Autodesk Inventor part; units mm, degrees
(part 2 of 3)
  line L936 (44.1495, 7.0872) -> (44.0754, 6.988)
  line L937 (44.0754, 6.988) -> (43.9994, 6.8902)
  line L938 (43.9994, 6.8902) -> (43.7335, 6.2149)
  line L939 (43.7335, 6.2149) -> (43.6108, 5.2944)
  line L940 (43.6108, 5.2944) -> (43.608, 5.0726)
  line L941 (43.608, 5.0726) -> (42.6667, 5.0726)
  line L942 (42.6667, 5.0726) -> (42.6667, 8.4846)
  line L943 (42.6667, 8.4846) -> (50.4254, 8.4846)
  line L944 (50.4254, 8.4846) -> (50.4254, 5.0726)
  line L945 (50.4254, 5.0726) -> (49.484, 5.0726)
  line L946 (49.484, 5.0726) -> (49.4812, 5.2903)
  line L947 (49.4812, 5.2903) -> (49.3613, 6.2039)
  line L948 (49.3613, 6.2039) -> (49.0967, 6.8806)
  line L949 (49.0967, 6.8806) -> (49.0223, 6.9798)
  line L950 (49.0223, 6.9798) -> (48.9466, 7.0804)
  line L951 (48.9466, 7.0804) -> (48.4381, 7.429)
  line L952 (48.4381, 7.429) -> (47.8013, 7.5792)
  line L953 (47.8013, 7.5792) -> (47.5889, 7.5792)
  line L954 (47.5889, 7.5792) -> (47.4088, 7.5792)
  line L955 (47.4088, 7.5792) -> (47.4088, 1.943)
  line L956 (47.4088, 1.943) -> (47.4088, 1.7859)
  line L957 (47.4088, 1.7859) -> (47.5204, 1.3353)
  line L958 (47.5204, 1.3353) -> (47.544, 1.3133)
  line L959 (47.544, 1.3133) -> (47.5658, 1.2912)
  line L960 (47.5658, 1.2912) -> (48.0631, 1.181)
  line L961 (48.0631, 1.181) -> (48.23, 1.181)
  line L962 (48.23, 1.181) -> (48.9313, 1.181)
  line L963 (48.9313, 1.181) -> (48.9313, 0.2453)
  line L964 (48.9313, 0.2453) -> (44.1536, 0.2453)
  line L965 (44.1536, 0.2453) -> (44.1536, 1.181)
  line L966 (44.1536, 1.181) -> (44.8663, 1.181)
  line L967 (44.8663, 1.181) -> (45.0357, 1.181)
  line L968 (45.0357, 1.181) -> (45.5221, 1.2898)
  line L969 (45.5221, 1.2898) -> (45.5442, 1.3105)
  line L970 (45.5442, 1.3105) -> (45.5661, 1.3326)
  line L971 (45.5661, 1.3326) -> (45.6766, 1.7915)
  line L972 (45.6766, 1.7915) -> (45.6766, 1.943)
  line L973 (45.6766, 1.943) -> (45.6766, 7.5792)
  line L974 (52.4548, 0.2453) -> (52.4548, 1.181)
  line L975 (52.4548, 1.181) -> (52.9361, 1.181)
  line L976 (52.9361, 1.181) -> (53.104, 1.181)
  line L977 (53.104, 1.181) -> (53.5904, 1.2898)
  line L978 (53.5904, 1.2898) -> (53.6128, 1.3105)
  line L979 (53.6128, 1.3105) -> (53.6346, 1.3326)
  line L980 (53.6346, 1.3326) -> (53.7449, 1.7915)
  line L981 (53.7449, 1.7915) -> (53.7449, 1.943)
  line L982 (53.7449, 1.943) -> (53.7449, 6.7937)
  line L983 (53.7449, 6.7937) -> (53.7449, 6.9522)
  line L984 (53.7449, 6.9522) -> (53.6346, 7.4056)
  line L985 (53.6346, 7.4056) -> (53.6128, 7.4262)
  line L986 (53.6128, 7.4262) -> (53.5904, 7.4483)
  line L987 (53.5904, 7.4483) -> (53.0987, 7.5544)
  line L988 (53.0987, 7.5544) -> (52.9361, 7.5544)
  line L989 (52.9361, 7.5544) -> (52.4548, 7.5544)
  line L990 (52.4548, 7.5544) -> (52.4548, 8.4846)
  line L991 (52.4548, 8.4846) -> (60.5618, 8.4846)
  line L992 (60.5618, 8.4846) -> (60.5618, 5.2047)
  line L993 (60.5618, 5.2047) -> (59.6263, 5.2047)
  line L994 (59.6263, 5.2047) -> (59.6192, 5.4403)
  line L995 (59.6192, 5.4403) -> (59.494, 6.3788)
  line L996 (59.494, 6.3788) -> (59.2375, 7.0058)
  line L997 (59.2375, 7.0058) -> (59.1674, 7.0843)
  line L998 (59.1674, 7.0843) -> (59.0973, 7.1629)
  line L999 (59.0973, 7.1629) -> (58.5278, 7.4371)
  line L1000 (58.5278, 7.4371) -> (57.7231, 7.5543)
  line L1001 (57.7231, 7.5543) -> (57.4557, 7.5543)
  line L1002 (57.4557, 7.5543) -> (55.477, 7.5543)
  line L1003 (55.477, 7.5543) -> (55.477, 5.0242)
  line L1004 (55.477, 5.0242) -> (55.9454, 5.0242)
  line L1005 (55.9454, 5.0242) -> (56.1054, 5.0242)
  line L1006 (56.1054, 5.0242) -> (56.5847, 5.0917)
  line L1007 (56.5847, 5.0917) -> (56.9184, 5.2474)
  line L1008 (56.9184, 5.2474) -> (56.9583, 5.2915)
  line L1009 (56.9583, 5.2915) -> (56.9982, 5.337)
  line L1010 (56.9982, 5.337) -> (57.1526, 5.7311)
  line L1011 (57.1526, 5.7311) -> (57.2476, 6.3581)
  line L1012 (57.2476, 6.3581) -> (57.2588, 6.518)
  line L1013 (57.2588, 6.518) -> (58.193, 6.5235)
  line L1014 (58.193, 6.5235) -> (58.193, 2.3921)
  line L1015 (58.193, 2.3921) -> (57.2588, 2.399)
  line L1016 (57.2588, 2.399) -> (57.2489, 2.5768)
  line L1017 (57.2489, 2.5768) -> (57.1569, 3.2727)
  line L1018 (57.1569, 3.2727) -> (57.0038, 3.7178)
  line L1019 (57.0038, 3.7178) -> (56.9639, 3.7688)
  line L1020 (56.9639, 3.7688) -> (56.9238, 3.8211)
  line L1021 (56.9238, 3.8211) -> (56.5918, 4.0003)
  line L1022 (56.5918, 4.0003) -> (56.1148, 4.0775)
  line L1023 (56.1148, 4.0775) -> (55.9563, 4.0775)
  line L1024 (55.9563, 4.0775) -> (55.477, 4.0775)
  line L1025 (55.477, 4.0775) -> (55.477, 1.1808)
  line L1026 (55.477, 1.1808) -> (57.6362, 1.1808)
  line L1027 (57.6362, 1.1808) -> (57.8636, 1.1808)
  line L1028 (57.8636, 1.1808) -> (58.5458, 1.3062)
  line L1029 (58.5458, 1.3062) -> (59.0487, 1.5998)
  line L1030 (59.0487, 1.5998) -> (59.1163, 1.6825)
  line L1031 (59.1163, 1.6825) -> (59.1826, 1.7665)
  line L1032 (59.1826, 1.7665) -> (59.4442, 2.4459)
  line L1033 (59.4442, 2.4459) -> (59.6083, 3.4767)
  line L1034 (59.6083, 3.4767) -> (59.6263, 3.7357)
  line L1035 (59.6263, 3.7357) -> (60.562, 3.7357)
  line L1036 (60.562, 3.7357) -> (60.562, 0.2453)
  line L1037 (60.562, 0.2453) -> (52.4548, 0.2453)
  line L1038 (69.1459, 3.4353) -> (70.2, 3.4353)
  line L1039 (70.2, 3.4353) -> (70.1798, 3.1625)
  line L1040 (70.1798, 3.1625) -> (69.8872, 1.9801)
  line L1041 (69.8872, 1.9801) -> (69.3375, 1.0459)
  line L1042 (69.3375, 1.0459) -> (69.1899, 0.8957)
  line L1043 (69.1899, 0.8957) -> (69.041, 0.7469)
  line L1044 (69.041, 0.7469) -> (68.1426, 0.2246)
  line L1045 (68.1426, 0.2246) -> (67.1215, 0)
  line L1046 (67.1215, 0) -> (66.7827, 0)
  line L1047 (66.7827, 0) -> (66.3735, 0)
  line L1048 (66.3735, 0) -> (65.2668, 0.2356)
  line L1049 (65.2668, 0.2356) -> (65.1454, 0.2825)
  line L1050 (65.1454, 0.2825) -> (65.0225, 0.3294)
  line L1051 (65.0225, 0.3294) -> (63.9338, 1.0487)
  line L1052 (63.9338, 1.0487) -> (63.8391, 1.1451)
  line L1053 (63.8391, 1.1451) -> (63.7329, 1.2513)
  line L1054 (63.7329, 1.2513) -> (62.931, 2.4626)
  line L1055 (62.931, 2.4626) -> (62.8769, 2.599)
  line L1056 (62.8769, 2.599) -> (62.8221, 2.7368)
  line L1057 (62.8221, 2.7368) -> (62.5508, 3.9632)
  line L1058 (62.5508, 3.9632) -> (62.5508, 4.3711)
  line L1059 (62.5508, 4.3711) -> (62.5508, 4.808)
  line L1060 (62.5508, 4.808) -> (62.8139, 5.9862)
  line L1061 (62.8139, 5.9862) -> (62.8675, 6.1185)
  line L1062 (62.8675, 6.1185) -> (62.9196, 6.2522)
  line L1063 (62.9196, 6.2522) -> (63.7192, 7.4483)
  line L1064 (63.7192, 7.4483) -> (63.8266, 7.5544)
  line L1065 (63.8266, 7.5544) -> (63.9229, 7.6522)
  line L1066 (63.9229, 7.6522) -> (65.0075, 8.384)
  line L1067 (65.0075, 8.384) -> (65.1274, 8.4336)
  line L1068 (65.1274, 8.4336) -> (65.2473, 8.4832)
  line L1069 (65.2473, 8.4832) -> (66.3179, 8.7299)
  line L1070 (66.3179, 8.7299) -> (66.675, 8.7299)
  line L1071 (66.675, 8.7299) -> (66.9851, 8.7299)
  line L1072 (66.9851, 8.7299) -> (67.8216, 8.5576)
  line L1073 (67.8216, 8.5576) -> (67.9193, 8.5232)
  line L1074 (67.9193, 8.5232) -> (68.0159, 8.4887)
  line L1075 (68.0159, 8.4887) -> (68.9737, 7.9568)
  line L1076 (68.9737, 7.9568) -> (69.0672, 7.8852)
  line L1077 (69.0672, 7.8852) -> (69.3128, 8.6224)
  line L1078 (69.3128, 8.6224) -> (70.2, 8.6224)
  line L1079 (70.2, 8.6224) -> (70.2, 5.2461)
  line L1080 (70.2, 5.2461) -> (69.2533, 5.2461)
  line L1081 (69.2533, 5.2461) -> (69.2284, 5.4431)
  line L1082 (69.2284, 5.4431) -> (68.9912, 6.2948)
  line L1083 (68.9912, 6.2948) -> (68.5959, 6.9672)
  line L1084 (68.5959, 6.9672) -> (68.4938, 7.0747)
  line L1085 (68.4938, 7.0747) -> (68.3905, 7.1836)
  line L1086 (68.3905, 7.1836) -> (67.7897, 7.5612)
  line L1087 (67.7897, 7.5612) -> (67.1283, 7.7224)
  line L1088 (67.1283, 7.7224) -> (66.9091, 7.7224)
  line L1089 (66.9091, 7.7224) -> (66.6556, 7.7224)
  line L1090 (66.6556, 7.7224) -> (65.8977, 7.4964)
  line L1091 (65.8977, 7.4964) -> (65.2378, 6.9686)
  line L1092 (65.2378, 6.9686) -> (65.1316, 6.817)
  line L1093 (65.1316, 6.817) -> (65.0239, 6.6668)
  line L1094 (65.0239, 6.6668) -> (64.6478, 5.738)
  line L1095 (64.6478, 5.738) -> (64.4867, 4.6673)
  line L1096 (64.4867, 4.6673) -> (64.4867, 4.3104)
  line L1097 (64.4867, 4.3104) -> (64.4867, 3.9741)
  line L1098 (64.4867, 3.9741) -> (64.6465, 2.9613)
  line L1099 (64.6465, 2.9613) -> (65.0202, 2.0972)
  line L1100 (65.0202, 2.0972) -> (65.1273, 1.9581)
  line L1101 (65.1273, 1.9581) -> (65.2335, 1.8203)
  line L1102 (65.2335, 1.8203) -> (65.8992, 1.3352)
  line L1103 (65.8992, 1.3352) -> (66.6734, 1.1271)
  line L1104 (66.6734, 1.1271) -> (66.9325, 1.1271)
  line L1105 (66.9325, 1.1271) -> (67.1367, 1.1271)
  line L1106 (67.1367, 1.1271) -> (67.7512, 1.2759)
  line L1107 (67.7512, 1.2759) -> (68.3067, 1.6204)
  line L1108 (68.3067, 1.6204) -> (68.4019, 1.7183)
  line L1109 (68.4019, 1.7183) -> (68.4954, 1.8175)
  line L1110 (68.4954, 1.8175) -> (68.8688, 2.4431)
  line L1111 (68.8688, 2.4431) -> (69.1154, 3.2479)
  line L1112 (69.1154, 3.2479) -> (69.1459, 3.4353)
  line L1113 (71.6716, 0.2452) -> (71.6716, 1.1809)
  line L1114 (71.6716, 1.1809) -> (72.1512, 1.1809)
  line L1115 (72.1512, 1.1809) -> (72.3193, 1.1809)
  line L1116 (72.3193, 1.1809) -> (72.8057, 1.2897)
  line L1117 (72.8057, 1.2897) -> (72.8278, 1.3104)
  line L1118 (72.8278, 1.3104) -> (72.8499, 1.3325)
  line L1119 (72.8499, 1.3325) -> (72.9599, 1.7914)
  line L1120 (72.9599, 1.7914) -> (72.9599, 1.9429)
  line L1121 (72.9599, 1.9429) -> (72.9599, 6.7936)
  line L1122 (72.9599, 6.7936) -> (72.9599, 6.9521)
  line L1123 (72.9599, 6.9521) -> (72.8499, 7.4055)
  line L1124 (72.8499, 7.4055) -> (72.8278, 7.4262)
  line L1125 (72.8278, 7.4262) -> (72.8058, 7.4482)
  line L1126 (72.8058, 7.4482) -> (72.3138, 7.5543)
  line L1127 (72.3138, 7.5543) -> (72.1512, 7.5543)
  line L1128 (72.1512, 7.5543) -> (71.6716, 7.5543)
  line L1129 (71.6716, 7.5543) -> (71.6716, 8.4845)
  line L1130 (71.6716, 8.4845) -> (76.09, 8.4845)
  line L1131 (76.09, 8.4845) -> (76.09, 7.5543)
  line L1132 (76.09, 7.5543) -> (75.5152, 7.5543)
  line L1133 (75.5152, 7.5543) -> (75.3427, 7.5543)
  line L1134 (75.3427, 7.5543) -> (74.8494, 7.4441)
  line L1135 (74.8494, 7.4441) -> (74.8273, 7.4221)
  line L1136 (74.8273, 7.4221) -> (74.804, 7.4014)
  line L1137 (74.804, 7.4014) -> (74.6935, 6.9466)
  line L1138 (74.6935, 6.9466) -> (74.6935, 6.7936)
  line L1139 (74.6935, 6.7936) -> (74.6935, 4.9705)
  line L1140 (74.6935, 4.9705) -> (78.2546, 4.9705)
  line L1141 (78.2546, 4.9705) -> (78.2546, 6.7936)
  line L1142 (78.2546, 6.7936) -> (78.2546, 6.9521)
  line L1143 (78.2546, 6.9521) -> (78.1446, 7.4055)
  line L1144 (78.1446, 7.4055) -> (78.1223, 7.4262)
  line L1145 (78.1223, 7.4262) -> (78.1005, 7.4482)
  line L1146 (78.1005, 7.4482) -> (77.6082, 7.5543)
  line L1147 (77.6082, 7.5543) -> (77.4456, 7.5543)
  line L1148 (77.4456, 7.5543) -> (76.8642, 7.5543)
  line L1149 (76.8642, 7.5543) -> (76.8642, 8.4845)
  line L1150 (76.8642, 8.4845) -> (81.2889, 8.4845)
  line L1151 (81.2889, 8.4845) -> (81.2889, 7.5545)
  line L1152 (81.2889, 7.5545) -> (80.8081, 7.5545)
  line L1153 (80.8081, 7.5545) -> (80.6357, 7.5545)
  line L1154 (80.6357, 7.5545) -> (80.1439, 7.4443)
  line L1155 (80.1439, 7.4443) -> (80.1216, 7.4222)
  line L1156 (80.1216, 7.4222) -> (80.0984, 7.4016)
  line L1157 (80.0984, 7.4016) -> (79.9864, 6.9468)
  line L1158 (79.9864, 6.9468) -> (79.9864, 6.7938)
  line L1159 (79.9864, 6.7938) -> (79.9864, 1.9431)
  line L1160 (79.9864, 1.9431) -> (79.9864, 1.786)
  line L1161 (79.9864, 1.786) -> (80.0984, 1.3354)
  line L1162 (80.0984, 1.3354) -> (80.1215, 1.3134)
  line L1163 (80.1215, 1.3134) -> (80.1439, 1.2913)
  line L1164 (80.1439, 1.2913) -> (80.6412, 1.1811)
  line L1165 (80.6412, 1.1811) -> (80.8081, 1.1811)
  line L1166 (80.8081, 1.1811) -> (81.2885, 1.1811)
  line L1167 (81.2885, 1.1811) -> (81.2885, 0.2452)
  line L1168 (81.2885, 0.2452) -> (76.8641, 0.2452)
  line L1169 (76.8641, 0.2452) -> (76.8641, 1.1809)
  line L1170 (76.8641, 1.1809) -> (77.4455, 1.1809)
  line L1171 (77.4455, 1.1809) -> (77.6139, 1.1809)
  line L1172 (77.6139, 1.1809) -> (78.1003, 1.2897)
  line L1173 (78.1003, 1.2897) -> (78.1222, 1.3104)
  line L1174 (78.1222, 1.3104) -> (78.1445, 1.3325)
  line L1175 (78.1445, 1.3325) -> (78.2545, 1.7914)
  line L1176 (78.2545, 1.7914) -> (78.2545, 1.9429)
  line L1177 (78.2545, 1.9429) -> (78.2545, 3.9811)
  line L1178 (78.2545, 3.9811) -> (74.6934, 3.9811)
  line L1179 (74.6934, 3.9811) -> (74.6934, 1.9429)
  line L1180 (74.6934, 1.9429) -> (74.6934, 1.7858)
  line L1181 (74.6934, 1.7858) -> (74.8039, 1.3352)
  line L1182 (74.8039, 1.3352) -> (74.8273, 1.3132)
  line L1183 (74.8273, 1.3132) -> (74.8494, 1.2911)
  line L1184 (74.8494, 1.2911) -> (75.3483, 1.1809)
  line L1185 (75.3483, 1.1809) -> (75.5151, 1.1809)
  line L1186 (75.5151, 1.1809) -> (76.0899, 1.1809)
  line L1187 (76.0899, 1.1809) -> (76.0899, 0.2452)
  line L1188 (76.0899, 0.2452) -> (71.6716, 0.2452)
  line L1189 (52.6024, 13.2512) -> (52.6024, 11.5604)
  line L1190 (52.6024, 11.5604) -> (45.3182, 11.5604)
  line L1191 (45.3182, 11.5604) -> (45.3182, 13.2512)
  line L1192 (53.6649, 13.2513) -> (53.6649, 11.5604)
  line L1193 (60.8501, 11.5604) -> (53.6649, 11.5604)
  line L1194 (60.8501, 11.5604) -> (60.8501, 13.2513)
  line L1195 (44.5216, 13.2512) -> (44.5216, 11.5604)
  line L1196 (44.5216, 11.5604) -> (37.3352, 11.5604)
  line L1197 (37.3352, 13.2512) -> (37.3352, 11.5604)
  line L1198 (28.9885, 13.2512) -> (28.9885, 11.5604)
  line L1199 (28.9885, 11.5604) -> (36.274, 11.5604)
  line L1200 (36.274, 11.5604) -> (36.274, 13.2512)
  point P0 (0, 0)
  point P1 (61.851, 32.2513)
  point P2 (69.27, 69.4749)
  point P3 (76.8568, 60.7794)
  point P4 (55.9435, 44.6898)
  point P5 (55.7616, 44.2764)
  point P6 (55.3607, 43.7411)
  point P7 (54.8184, 43.4358)
  point P8 (54.2073, 43.4068)
  point P9 (53.5699, 43.595)
  point P10 (52.949, 43.9402)
  point P11 (52.3875, 44.3812)
  point P12 (51.9728, 44.7946)
  point P13 (51.4497, 45.5014)
  point P14 (50.4445, 47.1945)
  point P15 (48.9872, 50.1931)
  point P16 (47.7848, 53.5182)
  point P17 (47.124, 56.1909)
  point P18 (59.2018, 36.8363)
  point P19 (59.6704, 36.454)
  point P20 (60.4793, 35.9702)
  point P21 (60.9796, 35.7697)
  constraints: 2402 end point, 447 parallel, 180 horizontal, 132 vertical, 69 perpendicular, 21 midpoint, 20 coincident, 8 collinear, 2068 other
extrude "Extrusion1" add sketch "Sketch1" against normal blind 25.4
sketch "Sketch3" plane through (0, 0, 0) normal (0, 0, 1) x (1, 0, 0)
  line L0 (24.3775, 20.4997) -> (24.5828, 19.3435) construction
  line L1 (24.5828, 19.3435) -> (24.6021, 19.0679) construction
  line L2 (24.6021, 19.0679) -> (19.5516, 19.0679) construction
  line L3 (19.5516, 19.0679) -> (19.5888, 19.3298) construction
  line L4 (19.5888, 19.3298) -> (19.892, 20.4459) construction
  line L5 (19.892, 20.4459) -> (20.355, 21.31) construction
  line L6 (20.355, 21.31) -> (20.4721, 21.4437) construction
  line L7 (20.4721, 21.4437) -> (20.5879, 21.5787) construction
  line L8 (20.5879, 21.5787) -> (21.2728, 22.0514) construction
  line L9 (21.2728, 22.0514) -> (22.0279, 22.2526) construction
  line L10 (22.0279, 22.2526) -> (22.5185, 22.2526) construction
  line L11 (22.5185, 22.2526) -> (23.2351, 22.0624) construction
  line L12 (23.2351, 22.0624) -> (23.8345, 21.6145) construction
  line L13 (23.8345, 21.6145) -> (23.9282, 21.4864) construction
  line L14 (23.9282, 21.4864) -> (24.022, 21.3596) construction
  line L15 (24.022, 21.3596) -> (24.3775, 20.4997) construction
  line L16 (25.7492, 15.8331) -> (27.8727, 15.8331) construction
  line L17 (25.6969, 15.5906) -> (25.7492, 15.8331) construction
  line L18 (25.3304, 14.5846) -> (25.6969, 15.5906) construction
  line L19 (24.8178, 13.8569) -> (25.3304, 14.5846) construction
  line L20 (24.6937, 13.7522) -> (24.8178, 13.8569) construction
  line L21 (24.5684, 13.6489) -> (24.6937, 13.7522) construction
  line L22 (23.7677, 13.2865) -> (24.5684, 13.6489) construction
  line L23 (22.8086, 13.1294) -> (23.7677, 13.2865) construction
  line L24 (22.1747, 13.1294) -> (22.8086, 13.1294) construction
  line L25 (21.228, 13.3954) -> (22.1747, 13.1294) construction
  line L26 (20.4162, 14.014) -> (21.228, 13.3954) construction
  line L27 (20.2853, 14.1904) -> (20.4162, 14.014) construction
  line L28 (20.1544, 14.3682) -> (20.2853, 14.1904) construction
  line L29 (19.6789, 15.494) -> (20.1544, 14.3682) construction
  line L30 (19.4389, 16.9409) -> (19.6789, 15.494) construction
  line L31 (19.4279, 17.2771) -> (19.4389, 16.9409) construction
  line L32 (27.9479, 17.2771) -> (19.4279, 17.2771) construction
  line L33 (27.9479, 17.6601) -> (27.9479, 17.2771) construction
  line L34 (27.8569, 18.8102) -> (27.9479, 17.6601) construction
  line L35 (27.5856, 20.1496) -> (27.8569, 18.8102) construction
  line L36 (27.1351, 21.2948) -> (27.5856, 20.1496) construction
  line L37 (26.6857, 22.0307) -> (27.1351, 21.2948) construction
  line L38 (26.5039, 22.247) -> (26.6857, 22.0307) construction
  line L39 (26.3273, 22.4551) -> (26.5039, 22.247) construction
  line L40 (25.699, 22.9953) -> (26.3273, 22.4551) construction
  line L41 (24.7303, 23.53) -> (25.699, 22.9953) construction
  line L42 (23.5989, 23.8497) -> (24.7303, 23.53) construction
  line L43 (22.6274, 23.9558) -> (23.5989, 23.8497) construction
  line L44 (21.9645, 23.9558) -> (22.6274, 23.9558) construction
  line L45 (20.9476, 23.8456) -> (21.9645, 23.9558) construction
  line L46 (19.7321, 23.5134) -> (20.9476, 23.8456) construction
  line L47 (18.6545, 22.9609) -> (19.7321, 23.5134) construction
  line L48 (17.9297, 22.4014) -> (18.6545, 22.9609) construction
  line L49 (17.7188, 22.185) -> (17.9297, 22.4014) construction
  line L50 (17.5066, 21.9687) -> (17.7188, 22.185) construction
  line L51 (16.9581, 21.2301) -> (17.5066, 21.9687) construction
  line L52 (16.4166, 20.1345) -> (16.9581, 21.2301) construction
  line L53 (16.0914, 18.8998) -> (16.4166, 20.1345) construction
  line L54 (15.9839, 17.869) -> (16.0914, 18.8998) construction
  line L55 (15.9839, 17.1772) -> (15.9839, 17.869) construction
  line L56 (16.09, 16.1355) -> (15.9839, 17.1772) construction
  line L57 (16.4124, 14.8925) -> (16.09, 16.1355) construction
  line L58 (16.9485, 13.7983) -> (16.4124, 14.8925) construction
  line L59 (17.4887, 13.0652) -> (16.9485, 13.7983) construction
  line L60 (17.6995, 12.8502) -> (17.4887, 13.0652) construction
  line L61 (17.909, 12.638) -> (17.6995, 12.8502) construction
  line L62 (18.6297, 12.0868) -> (17.909, 12.638) construction
  line L63 (19.7087, 11.541) -> (18.6297, 12.0868) construction
  line L64 (20.9338, 11.2145) -> (19.7087, 11.541) construction
  line L65 (21.9618, 11.1042) -> (20.9338, 11.2145) construction
  line L66 (22.8327, 11.1042) -> (21.9618, 11.1042) construction
  line L67 (24.4174, 11.4214) -> (22.8327, 11.1042) construction
  line L68 (25.8657, 12.1589) -> (24.4174, 11.4214) construction
  line L69 (26.1135, 12.3698) -> (25.8657, 12.1589) construction
  line L70 (26.3617, 12.5807) -> (26.1135, 12.3698) construction
  line L71 (27.2972, 13.8693) -> (26.3617, 12.5807) construction
  line L72 (27.8273, 15.4679) -> (27.2972, 13.8693) construction
  line L73 (27.8727, 15.8331) -> (27.8273, 15.4679) construction
  line L74 (19.5516, 19.0679) -> (24.6021, 19.0679) construction
  line L75 (27.9479, 17.2771) -> (19.4279, 17.2771)
  line L76 (25.7492, 15.8331) -> (27.8727, 15.8331)
  line L77 (25.7492, 15.8331) -> (27.8727, 15.8331) construction
  line L78 (24.6021, 19.0679) -> (19.5516, 19.0679) construction
  line L79 (24.5828, 19.3435) -> (24.6021, 19.0679) construction
  line L80 (19.5888, 19.3298) -> (19.5516, 19.0679) construction
  line L81 (19.892, 20.4459) -> (19.5888, 19.3298) construction
  line L82 (19.892, 20.4459) -> (20.355, 21.31) construction
  line L83 (22.0279, 22.2526) -> (21.2728, 22.0514) construction
  line L84 (23.2351, 22.0624) -> (23.8345, 21.6145) construction
  line L85 (23.9282, 21.4864) -> (24.022, 21.3596) construction
  line L86 (24.022, 21.3596) -> (24.3775, 20.4997) construction
  line L87 (24.3775, 20.4997) -> (24.5828, 19.3435) construction
  spline S0 degree 4 poles (19.5516, 19.0679) (19.5728, 19.217) (19.5818, 19.3523) (19.7782, 20.4265) (20.3812, 21.3604) (20.4936, 21.524) (21.2694, 22.1484) (22.0473, 22.2766) (22.4831, 22.2706) (23.2309, 22.1723) (23.9246, 21.5537) (24.0363, 21.3665) (24.6968, 19.922) (24.5548, 19.1799) (24.6021, 19.0679) knots 0 0 0 0 0 0.111145 0.186515 0.271328 0.351598 0.424995 0.504672 0.583231 0.654159 0.731357 0.813837 1 1 1 1 1
  line L88 (19.5516, 19.0679) -> (19.5888, 19.3298) construction
  line L89 (27.8727, 15.8331) -> (27.8273, 15.4679) construction
  line L90 (27.9479, 17.6601) -> (27.9479, 17.2771) construction
  line L91 (27.8569, 18.8102) -> (27.9479, 17.6601) construction
  line L92 (27.5856, 20.1496) -> (27.8569, 18.8102) construction
  line L93 (26.6857, 22.0307) -> (27.1351, 21.2948) construction
  line L94 (26.5039, 22.247) -> (26.6857, 22.0307) construction
  line L95 (26.3273, 22.4551) -> (26.5039, 22.247) construction
  line L96 (25.699, 22.9953) -> (26.3273, 22.4551) construction
  line L97 (24.7303, 23.53) -> (25.699, 22.9953) construction
  line L98 (23.5989, 23.8497) -> (24.7303, 23.53) construction
  line L99 (22.6274, 23.9558) -> (23.5989, 23.8497) construction
  line L100 (21.9645, 23.9558) -> (22.6274, 23.9558) construction
  line L101 (20.9476, 23.8456) -> (21.9645, 23.9558) construction
  line L102 (19.7321, 23.5134) -> (20.9476, 23.8456) construction
  line L103 (18.6545, 22.9609) -> (19.7321, 23.5134) construction
  line L104 (17.7188, 22.185) -> (17.9297, 22.4014) construction
  line L105 (16.9581, 21.2301) -> (17.5066, 21.9687) construction
  line L106 (16.0914, 18.8998) -> (16.4166, 20.1345) construction
  line L107 (15.9839, 17.869) -> (16.0914, 18.8998) construction
  line L108 (15.9839, 17.1772) -> (15.9839, 17.869) construction
  line L109 (16.09, 16.1355) -> (15.9839, 17.1772) construction
  line L110 (16.4124, 14.8925) -> (16.09, 16.1355) construction
  line L111 (16.9485, 13.7983) -> (16.4124, 14.8925) construction
  line L112 (17.4887, 13.0652) -> (16.9485, 13.7983) construction
  line L113 (17.909, 12.638) -> (17.6995, 12.8502) construction
  line L114 (18.6297, 12.0868) -> (17.909, 12.638) construction
  line L115 (19.7087, 11.541) -> (18.6297, 12.0868) construction
  line L116 (20.9338, 11.2145) -> (19.7087, 11.541) construction
  line L117 (22.8327, 11.1042) -> (21.9618, 11.1042) construction
  line L118 (24.4174, 11.4214) -> (22.8327, 11.1042) construction
  line L119 (26.1135, 12.3698) -> (25.8657, 12.1589) construction
  line L120 (26.3617, 12.5807) -> (26.1135, 12.3698) construction
  line L121 (27.2972, 13.8693) -> (26.3617, 12.5807) construction
  line L122 (27.8273, 15.4679) -> (27.2972, 13.8693) construction
  spline S1 degree 4 poles (27.9479, 17.2771) (27.9479, 17.4772) (27.9632, 17.7095) (27.8822, 18.9432) (27.6296, 20.1068) (27.2882, 21.0633) (26.764, 21.9883) (26.4896, 22.2358) (26.3127, 22.5219) (25.5238, 23.1665) (24.7279, 23.5751) (23.678, 23.8807) (22.6028, 23.9716) (21.9743, 23.9718) (20.8442, 23.8732) (19.7289, 23.5547) (18.8508, 23.1307) (17.9564, 22.4756) (17.7325, 22.1716) (17.432, 21.9386) (16.7903, 21.0274) (16.3749, 20.1358) (16.0629, 18.9956) (15.9676, 17.8518) (15.9687, 17.1928) (16.0613, 16.0392) (16.3692, 14.8946) (16.7815, 14.0024) (17.4136, 13.0963) (17.7129, 12.8622) (17.9362, 12.5656) (18.8303, 11.9156) (19.7068, 11.4955) (20.9046, 11.174) (22.0202, 11.0879) (22.8682, 11.0746) (24.2073, 11.2389) (25.8516, 12.0509) (26.0824, 12.398) (26.4697, 12.5892) (27.5378, 13.9993) (27.8494, 15.4193) (27.8461, 15.6195) (27.8727, 15.8331) knots 0 0 0 0 0 0.033657 0.059492 0.087341 0.111662 0.131775 0.150595 0.170216 0.193433 0.219682 0.245306 0.270666 0.296275 0.322613 0.349878 0.37414 0.394681 0.414302 0.43489 0.459253 0.486658 0.513234 0.539275 0.565337 0.591957 0.619374 0.643705 0.664215 0.683742 0.704214 0.728441 0.755731 0.782895 0.811175 0.840424 0.86677 0.890757 0.914682 0.938757 0.963067 1 1 1 1 1
  line L123 (27.8727, 15.8331) -> (27.8273, 15.4679) construction
  line L124 (19.4279, 17.2771) -> (19.4389, 16.9409) construction
  line L125 (19.4389, 16.9409) -> (19.6789, 15.494) construction
  line L126 (19.6789, 15.494) -> (20.1544, 14.3682) construction
  line L127 (20.1544, 14.3682) -> (20.2853, 14.1904) construction
  line L128 (20.4162, 14.014) -> (21.228, 13.3954) construction
  line L129 (21.228, 13.3954) -> (22.1747, 13.1294) construction
  line L130 (22.1747, 13.1294) -> (22.8086, 13.1294) construction
  line L131 (22.8086, 13.1294) -> (23.7677, 13.2865) construction
  line L132 (23.7677, 13.2865) -> (24.5684, 13.6489) construction
  line L133 (24.5684, 13.6489) -> (24.6937, 13.7522) construction
  line L134 (24.8178, 13.8569) -> (25.3304, 14.5846) construction
  line L135 (25.3304, 14.5846) -> (25.6969, 15.5906) construction
  line L136 (27.9479, 17.2771) -> (19.4279, 17.2771) projected
  line L137 (19.4279, 17.2771) -> (19.4334, 17.109) construction
  line L138 (19.4334, 17.109) -> (19.4389, 16.9409) construction
  line L139 (19.4389, 16.9409) -> (19.5589, 16.2174) construction
  line L140 (19.5589, 16.2174) -> (19.6789, 15.494) construction
  line L141 (19.6789, 15.494) -> (20.1544, 14.3682) construction
  line L142 (20.1544, 14.3682) -> (20.2853, 14.1904) construction
  line L143 (20.2853, 14.1904) -> (20.4162, 14.014) construction
  line L144 (20.4162, 14.014) -> (20.8221, 13.7047) construction
  line L145 (20.8221, 13.7047) -> (21.228, 13.3954) construction
  line L146 (21.228, 13.3954) -> (21.7013, 13.2624) construction
  line L147 (21.7013, 13.2624) -> (22.1747, 13.1294) construction
  line L148 (22.1747, 13.1294) -> (22.4916, 13.1294) construction
  line L149 (22.4916, 13.1294) -> (22.8086, 13.1294) construction
  line L150 (22.8086, 13.1294) -> (23.2881, 13.2079) construction
  line L151 (23.2881, 13.2079) -> (23.7677, 13.2865) construction
  line L152 (23.7677, 13.2865) -> (24.168, 13.4677) construction
  line L153 (24.168, 13.4677) -> (24.5684, 13.6489) construction
  line L154 (24.5684, 13.6489) -> (24.6937, 13.7522) construction
  line L155 (24.6937, 13.7522) -> (24.8178, 13.8569) construction
  line L156 (24.8178, 13.8569) -> (25.0741, 14.2208) construction
  line L157 (25.0741, 14.2208) -> (25.3304, 14.5846) construction
  line L158 (25.3304, 14.5846) -> (25.5137, 15.0876) construction
  line L159 (25.5137, 15.0876) -> (25.6969, 15.5906) construction
  line L160 (25.6969, 15.5906) -> (25.7492, 15.8331) projected
  line L161 (25.6969, 15.5906) -> (25.7492, 15.8331) construction
  spline S2 degree 4 poles (19.4279, 17.2771) (19.4334, 17.109) (19.4389, 16.9409) (19.5589, 16.2174) (19.6789, 15.494) (20.1544, 14.3682) (20.2853, 14.1904) (20.4162, 14.014) (20.8221, 13.7047) (21.228, 13.3954) (21.7013, 13.2624) (22.1747, 13.1294) (22.4916, 13.1294) (22.8086, 13.1294) (23.2881, 13.2079) (23.7677, 13.2865) (24.168, 13.4677) (24.5684, 13.6489) (24.6937, 13.7522) (24.8178, 13.8569) (25.0741, 14.2208) (25.3304, 14.5846) (25.5137, 15.0876) (25.6969, 15.5906) (25.7492, 15.8331) knots 1 1 1 1 1 2 3 4 5 6 7 8 9 10 11 12 13 14 15 16 17 18 19 20 21 22 22 22 22 22
  line L162 (19.4279, 17.2771) -> (27.9479, 17.2771)
  line L163 (27.8727, 15.8331) -> (25.7492, 15.8331)
  line L164 (19.5516, 19.0679) -> (24.6021, 19.0679)
  point P0 (0, 0)
  point P1 (19.9166, 14.9311)
  point P2 (24.168, 13.4677)
  constraints: 38 coincident, 14 end point, 13 collinear, 10 midpoint, 5 horizontal, 2 parallel, 1 vertical, 61 other
sketch "Sketch4" plane through (0, 0, 0) normal (0, 0, 1) x (1, 0, 0)
  line L0 (16.3578, 25.6719) -> (28.2265, 25.6719)
  line L1 (28.2265, 25.6719) -> (28.2265, 20.5919)
  line L2 (28.2265, 20.5919) -> (16.3578, 20.5919)
  line L3 (16.3578, 20.5919) -> (16.3578, 25.6719)
  line L4 (28.2265, 20.5919) -> (14.4599, 20.5919)
  line L5 (14.4599, 20.5919) -> (14.4599, 10.0882)
  line L6 (14.4599, 10.0882) -> (28.2265, 10.0882)
  line L7 (28.2265, 10.0882) -> (28.2265, 20.5919)
  line L8 (15.9768, 28.5255) -> (15.9768, 21.4991) projected
  line L9 (15.9839, 17.1772) -> (15.9839, 17.869) projected
  line L10 (22.8327, 11.1042) -> (21.9618, 11.1042) projected
  line L11 (28.9885, 13.2512) -> (28.9885, 11.5604) projected
  line L12 (24.6021, 19.0679) -> (19.5516, 19.0679) projected
  point P0 (0, 0)
  dimension "d2" = 0.381
  dimension "d3" = 1.524
  dimension "d4" = 1.016
  dimension "d5" = 0.762
  dimension "d6" = 1.524
  dimension "d7" = 5.08
  constraints: 16 end point, 4 parallel, 2 horizontal, 2 perpendicular
  measures "d2" distance between parallel lines of L8 L3
  measures "d3" distance between parallel lines of L9 L5
  measures "d4" distance between parallel lines of L10 L6
  measures "d5" distance between parallel lines of L11 L7
  measures "d6" distance between parallel lines of L12 L2
  measures "d7" distance between parallel lines of L4 L0
extrude "Extrusion2" cut sketch "Sketch4" against normal through all
extrude "Extrusion3" add sketch "Sketch3" against normal blind 25.4
sketch "Sketch5" plane through (0, 0, 0) normal (0, 0, 1) x (1, 0, 0)
  line L0 (107.191, 19.0679) -> (102.1405, 19.0679)
  spline S0 degree 4 poles (102.1405, 19.0679) (102.1617, 19.217) (102.1707, 19.3523) (102.367, 20.4265) (102.97, 21.3604) (103.0825, 21.524) (103.8582, 22.1484) (104.6362, 22.2766) (105.072, 22.2706) (105.8198, 22.1723) (106.5135, 21.5537) (106.6252, 21.3665) (107.2857, 19.922) (107.1436, 19.1799) (107.191, 19.0679) knots -1 -1 -1 -1 -1 -0.888855 -0.813485 -0.728672 -0.648402 -0.575005 -0.495328 -0.416769 -0.345841 -0.268643 -0.186163 0 0 0 0 0
  line L1 (110.4615, 15.8331) -> (108.3381, 15.8331)
  spline S1 degree 4 poles (108.3381, 15.8331) (108.2858, 15.5906) (108.1025, 15.0876) (107.9192, 14.5846) (107.663, 14.2208) (107.4067, 13.8569) (107.2826, 13.7522) (107.1572, 13.6489) (106.7569, 13.4677) (106.3565, 13.2865) (105.877, 13.208) (105.3974, 13.1294) (105.0805, 13.1294) (104.7635, 13.1294) (104.2902, 13.2624) (103.8168, 13.3954) (103.411, 13.7047) (103.0051, 14.014) (102.8742, 14.1904) (102.7432, 14.3682) (102.2677, 15.494) (102.1478, 16.2174) (102.0278, 16.9409) (102.0223, 17.109) (102.0167, 17.2771) knots 1 1 1 1 1 2 3 4 5 6 7 8 9 10 11 12 13 14 15 16 17 18 19 20 21 22 22 22 22 22
  line L2 (102.0167, 17.2771) -> (110.5368, 17.2771)
  spline S2 degree 4 poles (110.5368, 17.2771) (110.5368, 17.4773) (110.5521, 17.7095) (110.4711, 18.9432) (110.2184, 20.1068) (109.8771, 21.0633) (109.3529, 21.9883) (109.0785, 22.2358) (108.9016, 22.5219) (108.1127, 23.1665) (107.3168, 23.5751) (106.2669, 23.8807) (105.1916, 23.9716) (104.5631, 23.9718) (103.433, 23.8732) (102.3177, 23.5548) (101.4397, 23.1308) (100.5452, 22.4756) (100.3214, 22.1716) (100.0209, 21.9386) (99.3791, 21.0274) (98.9638, 20.1358) (98.6517, 18.9956) (98.5565, 17.8518) (98.5576, 17.1928) (98.6502, 16.0392) (98.958, 14.8946) (99.3704, 14.0024) (100.0024, 13.0964) (100.3017, 12.8622) (100.5251, 12.5656) (101.4191, 11.9156) (102.2956, 11.4955) (103.4934, 11.174) (104.6091, 11.0879) (105.4571, 11.0746) (106.7962, 11.2389) (108.4405, 12.0509) (108.6713, 12.398) (109.0586, 12.5892) (110.1267, 13.9993) (110.4383, 15.4193) (110.435, 15.6195) (110.4615, 15.8331) knots 0 0 0 0 0 0.033657 0.059492 0.087341 0.111662 0.131775 0.150595 0.170216 0.193433 0.219682 0.245306 0.270666 0.296275 0.322613 0.349878 0.37414 0.394681 0.414302 0.43489 0.459253 0.486658 0.513234 0.539275 0.565337 0.591957 0.619374 0.643705 0.664215 0.683742 0.704214 0.728441 0.755731 0.782895 0.811175 0.840424 0.86677 0.890757 0.914682 0.938757 0.963067 1 1 1 1 1
  line L3 (27.8727, 15.8331) -> (25.7492, 15.8331) projected
  line L4 (108.3384, 15.8331) -> (110.4615, 15.8331) projected
  line L5 (121.5423, 15.8329) -> (123.666, 15.8329) projected
  line L6 (120.3954, 19.0679) -> (115.3449, 19.0679)
  spline S3 degree 4 poles (115.3449, 19.0679) (115.3661, 19.217) (115.3752, 19.3523) (115.5715, 20.4265) (116.1745, 21.3604) (116.2869, 21.524) (117.0627, 22.1484) (117.8407, 22.2766) (118.2764, 22.2706) (119.0242, 22.1723) (119.7179, 21.5537) (119.8296, 21.3665) (120.4901, 19.922) (120.3481, 19.1799) (120.3954, 19.0679) knots -1 -1 -1 -1 -1 -0.888855 -0.813485 -0.728672 -0.648402 -0.575005 -0.495328 -0.416769 -0.345841 -0.268643 -0.186163 0 0 0 0 0
  line L7 (123.666, 15.8331) -> (121.5426, 15.8331)
  spline S4 degree 4 poles (121.5426, 15.8331) (121.4902, 15.5906) (121.307, 15.0876) (121.1237, 14.5846) (120.8674, 14.2208) (120.6111, 13.8569) (120.4871, 13.7522) (120.3617, 13.6489) (119.9613, 13.4677) (119.561, 13.2865) (119.0815, 13.208) (118.6019, 13.1294) (118.285, 13.1294) (117.968, 13.1294) (117.4946, 13.2624) (117.0213, 13.3954) (116.6154, 13.7047) (116.2095, 14.014) (116.0786, 14.1904) (115.9477, 14.3682) (115.4722, 15.494) (115.3522, 16.2174) (115.2323, 16.9409) (115.2267, 17.109) (115.2212, 17.2771) knots 1 1 1 1 1 2 3 4 5 6 7 8 9 10 11 12 13 14 15 16 17 18 19 20 21 22 22 22 22 22
  line L8 (115.2212, 17.2771) -> (123.7412, 17.2771)
  spline S5 degree 4 poles (123.7412, 17.2771) (123.7412, 17.4773) (123.7565, 17.7095) (123.6756, 18.9432) (123.4229, 20.1068) (123.0815, 21.0633) (122.5573, 21.9883) (122.283, 22.2358) (122.1061, 22.5219) (121.3171, 23.1665) (120.5212, 23.5751) (119.4713, 23.8807) (118.3961, 23.9716) (117.7676, 23.9718) (116.6375, 23.8732) (115.5222, 23.5548) (114.6442, 23.1308) (113.7497, 22.4756) (113.5258, 22.1716) (113.2253, 21.9386) (112.5836, 21.0274) (112.1683, 20.1358) (111.8562, 18.9956) (111.761, 17.8518) (111.762, 17.1928) (111.8547, 16.0392) (112.1625, 14.8946) (112.5749, 14.0024) (113.2069, 13.0964) (113.5062, 12.8622) (113.7295, 12.5656) (114.6236, 11.9156) (115.5001, 11.4955) (116.6979, 11.174) (117.8136, 11.0879) (118.6615, 11.0746) (120.0006, 11.2389) (121.6449, 12.0509) (121.8758, 12.398) (122.263, 12.5892) (123.3311, 13.9993) (123.6427, 15.4193) (123.6394, 15.6195) (123.666, 15.8331) knots 0 0 0 0 0 0.033657 0.059492 0.087341 0.111662 0.131775 0.150595 0.170216 0.193433 0.219682 0.245306 0.270666 0.296275 0.322613 0.349878 0.37414 0.394681 0.414302 0.43489 0.459253 0.486658 0.513234 0.539275 0.565337 0.591957 0.619374 0.643705 0.664215 0.683742 0.704214 0.728441 0.755731 0.782895 0.811175 0.840424 0.86677 0.890757 0.914682 0.938757 0.963067 1 1 1 1 1
  line L9 (73.0028, 17.2768) -> (64.4819, 17.2768) projected
  line L10 (69.657, 19.0679) -> (64.6065, 19.0679)
  spline S6 degree 4 poles (64.6065, 19.0679) (64.6277, 19.217) (64.6367, 19.3523) (64.8331, 20.4265) (65.4361, 21.3604) (65.5485, 21.524) (66.3243, 22.1484) (67.1022, 22.2766) (67.538, 22.2706) (68.2858, 22.1723) (68.9795, 21.5537) (69.0912, 21.3665) (69.7517, 19.922) (69.6097, 19.1799) (69.657, 19.0679) knots -1 -1 -1 -1 -1 -0.888855 -0.813485 -0.728672 -0.648402 -0.575005 -0.495328 -0.416769 -0.345841 -0.268643 -0.186163 0 0 0 0 0
  line L11 (72.9276, 15.8331) -> (70.8041, 15.8331)
  spline S7 degree 4 poles (70.8041, 15.8331) (70.7518, 15.5906) (70.5686, 15.0876) (70.3853, 14.5846) (70.129, 14.2208) (69.8727, 13.8569) (69.7486, 13.7522) (69.6233, 13.6489) (69.2229, 13.4677) (68.8226, 13.2865) (68.343, 13.208) (67.8635, 13.1294) (67.5465, 13.1294) (67.2296, 13.1294) (66.7562, 13.2624) (66.2829, 13.3954) (65.877, 13.7047) (65.4711, 14.014) (65.3402, 14.1904) (65.2093, 14.3682) (64.7338, 15.494) (64.6138, 16.2174) (64.4938, 16.9409) (64.4883, 17.109) (64.4828, 17.2771) knots 1 1 1 1 1 2 3 4 5 6 7 8 9 10 11 12 13 14 15 16 17 18 19 20 21 22 22 22 22 22
  line L12 (64.4828, 17.2771) -> (73.0028, 17.2771)
  spline S8 degree 4 poles (73.0028, 17.2771) (73.0028, 17.4773) (73.0181, 17.7095) (72.9371, 18.9432) (72.6845, 20.1068) (72.3431, 21.0633) (71.8189, 21.9883) (71.5445, 22.2358) (71.3676, 22.5219) (70.5787, 23.1665) (69.7828, 23.5751) (68.7329, 23.8807) (67.6577, 23.9716) (67.0292, 23.9718) (65.8991, 23.8732) (64.7838, 23.5548) (63.9057, 23.1308) (63.0113, 22.4756) (62.7874, 22.1716) (62.4869, 21.9386) (61.8452, 21.0274) (61.4298, 20.1358) (61.1178, 18.9956) (61.0225, 17.8518) (61.0236, 17.1928) (61.1162, 16.0392) (61.4241, 14.8946) (61.8364, 14.0024) (62.4685, 13.0964) (62.7678, 12.8622) (62.9911, 12.5656) (63.8852, 11.9156) (64.7617, 11.4955) (65.9595, 11.174) (67.0751, 11.0879) (67.9231, 11.0746) (69.2622, 11.2389) (70.9065, 12.0509) (71.1373, 12.398) (71.5246, 12.5892) (72.5927, 13.9993) (72.9043, 15.4193) (72.901, 15.6195) (72.9276, 15.8331) knots 0 0 0 0 0 0.033657 0.059492 0.087341 0.111662 0.131775 0.150595 0.170216 0.193433 0.219682 0.245306 0.270666 0.296275 0.322613 0.349878 0.37414 0.394681 0.414302 0.43489 0.459253 0.486658 0.513234 0.539275 0.565337 0.591957 0.619374 0.643705 0.664215 0.683742 0.704214 0.728441 0.755731 0.782895 0.811175 0.840424 0.86677 0.890757 0.914682 0.938757 0.963067 1 1 1 1 1
  point P0 (0, 0)
  point P1 (110.4615, 15.8331)
  point P2 (27.8727, 15.8331)
  point P3 (27.8727, 15.8331)
  point P4 (123.666, 15.8331)
  point P5 (72.9276, 15.8331)
  constraints: 18 end point, 30 other
sketch "Sketch6" plane through (0, 0, 0) normal (0, 0, 1) x (1, 0, 0)
  line L0 (98.3405, 36.6557) -> (128.8205, 36.6557)
  line L1 (128.8205, 36.6557) -> (128.8205, -1.5958)
  line L2 (128.8205, -1.5958) -> (98.3405, -1.5958)
  line L3 (98.3405, -1.5958) -> (98.3405, 36.6557)
  line L4 (104.5533, 23.9557) -> (105.2162, 23.9557) projected
  line L5 (105.4214, 11.1042) -> (104.5504, 11.1042) projected
  line L6 (123.7405, 17.6608) -> (123.7405, 17.2772) projected
  line L7 (73.0028, 17.2768) -> (64.4819, 17.2768) projected
  circle A0 centre (67.2569, 17.2768) radius 6.985
  point P0 (0, 0)
  dimension "d12" = 12.7
  dimension "d13" = 12.7
  dimension "d14" = 30.48
  dimension "d15" = 5.08
  dimension "d16" = 13.97
  dimension "d17" = 2.775
  constraints: 8 end point, 2 parallel, 1 centre point, 1 horizontal, 1 perpendicular, 1 point on line
  measures "d12" distance between parallel lines of L0 L4
  measures "d13" distance between parallel lines of L2 L5
  measures "d14" distance of L0.start L0.end
  measures "d15" distance between parallel lines of L1 L6
  measures "d16" diameter of A0
  measures "d17" distance of L7.end A0.centre
extrude "Extrusion4" cut sketch "Sketch6" against normal through all
extrude "Extrusion5" add sketch "Sketch5" against normal blind 25.4
sketch "Sketch7" plane through (0, 0, 0) normal (0, 0, 1) x (1, 0, 0)
  line L0 (63.7248, 41.0987) -> (64.7002, 37.0611) construction
  line L1 (64.7002, 37.0611) -> (64.5625, 36.9024) construction
  line L2 (64.5625, 36.9024) -> (63.8457, 36.2839) construction
  line L3 (63.8457, 36.2839) -> (63.0893, 35.88) construction
  line L4 (63.0893, 35.88) -> (62.9338, 35.8292) construction
  line L5 (62.9338, 35.8292) -> (61.9509, 40.717) construction
  line L6 (61.9509, 40.717) -> (61.0652, 35.7505) construction
  line L7 (61.0652, 35.7505) -> (60.894, 35.7889) construction
  line L8 (60.894, 35.7889) -> (60.0646, 36.1516) construction
  line L9 (60.0646, 36.1516) -> (59.2762, 36.7563) construction
  line L10 (59.2762, 36.7563) -> (59.1274, 36.9164) construction
  line L11 (59.1274, 36.9164) -> (60.1375, 41.0987) construction
  line L12 (60.1375, 41.0987) -> (58.1904, 38.2308) construction
  line L13 (58.1904, 38.2308) -> (58.0718, 38.4447) construction
  line L14 (58.0718, 38.4447) -> (57.5221, 39.6984) construction
  line L15 (57.5221, 39.6984) -> (57.0357, 41.2143) construction
  line L16 (57.0357, 41.2143) -> (56.9488, 41.5577) construction
  line L17 (56.9488, 41.5577) -> (55.9732, 44.7972) construction
  line L18 (55.9732, 44.7972) -> (55.9138, 44.5823) construction
  line L19 (55.9138, 44.5823) -> (55.6095, 43.9704) construction
  line L20 (55.6095, 43.9704) -> (55.1119, 43.5117) construction
  line L21 (55.1119, 43.5117) -> (54.5249, 43.3598) construction
  line L22 (54.5249, 43.3598) -> (53.8897, 43.4538) construction
  line L23 (53.8897, 43.4538) -> (53.2501, 43.7363) construction
  line L24 (53.2501, 43.7363) -> (52.6479, 44.1442) construction
  line L25 (52.6479, 44.1442) -> (52.1272, 44.6181) construction
  line L26 (52.1272, 44.6181) -> (51.8185, 44.971) construction
  line L27 (51.8185, 44.971) -> (51.7301, 45.0977) construction
  line L28 (51.7301, 45.0977) -> (51.1693, 45.9052) construction
  line L29 (51.1693, 45.9052) -> (49.7197, 48.4838) construction
  line L30 (49.7197, 48.4838) -> (48.2547, 51.9024) construction
  line L31 (48.2547, 51.9024) -> (47.3149, 55.134) construction
  line L32 (47.3149, 55.134) -> (46.9331, 57.2478) construction
  line L33 (46.9331, 57.2478) -> (46.8823, 57.9562) construction
  line L34 (46.8823, 57.9562) -> (46.8754, 57.8239) construction
  line L35 (46.8754, 57.8239) -> (46.845, 56.435) construction
  line L36 (46.845, 56.435) -> (46.8465, 56.2889) construction
  line L37 (46.8465, 56.2889) -> (46.8478, 55.5681) construction
  line L38 (46.8478, 55.5681) -> (47.147, 53.4045) construction
  line L39 (47.147, 53.4045) -> (48.0451, 49.9608) construction
  line L40 (48.0451, 49.9608) -> (49.5653, 46.2471) construction
  line L41 (49.5653, 46.2471) -> (51.1211, 43.4261) construction
  line L42 (51.1211, 43.4261) -> (51.7301, 42.5483) construction
  line L43 (51.7301, 42.5483) -> (51.8114, 42.431) construction
  line L44 (51.8114, 42.431) -> (52.0718, 42.0868) construction
  line L45 (52.0718, 42.0868) -> (52.528, 41.5369) construction
  line L46 (52.528, 41.5369) -> (53.0642, 40.9608) construction
  line L47 (53.0642, 40.9608) -> (53.6496, 40.4178) construction
  line L48 (53.6496, 40.4178) -> (54.2534, 39.973) construction
  line L49 (54.2534, 39.973) -> (54.8432, 39.686) construction
  line L50 (54.8432, 39.686) -> (55.3862, 39.6202) construction
  line L51 (55.3862, 39.6202) -> (55.7611, 39.7538) construction
  line L52 (55.7611, 39.7538) -> (55.8518, 39.8351) construction
  line L53 (55.8518, 39.8351) -> (55.8381, 39.7386) construction
  line L54 (55.8381, 39.7386) -> (55.5034, 38.7919) construction
  line L55 (55.5034, 38.7919) -> (55.4579, 38.7022) construction
  line L56 (55.4579, 38.7022) -> (53.5111, 34.8875) construction
  line L57 (53.5111, 34.8875) -> (53.5111, 38.0188) construction
  line L58 (53.5111, 38.0188) -> (53.4367, 38.0074) construction
  line L59 (53.4367, 38.0074) -> (52.6454, 37.9068) construction
  line L60 (52.6454, 37.9068) -> (52.5614, 37.8986) construction
  line L61 (52.5614, 37.8986) -> (52.3178, 37.875) construction
  line L62 (52.3178, 37.875) -> (50.9673, 37.7938) construction
  line L63 (50.9673, 37.7938) -> (49.567, 37.7592) construction
  line L64 (49.567, 37.7592) -> (49.1014, 37.7592) construction
  line L65 (49.1014, 37.7592) -> (49.1014, 32.2513) construction
  line L66 (49.1014, 32.2513) -> (74.6006, 32.2513) construction
  line L67 (74.6006, 32.2513) -> (74.6006, 37.7595) construction
  line L68 (74.6006, 37.7595) -> (74.1252, 37.7704) construction
  line L69 (74.1252, 37.7704) -> (72.1808, 37.841) construction
  line L70 (72.1808, 37.841) -> (70.8138, 37.9317) construction
  line L71 (70.8138, 37.9317) -> (70.6278, 37.9523) construction
  line L72 (70.6278, 37.9523) -> (70.5933, 37.9566) construction
  line L73 (70.5933, 37.9566) -> (70.2641, 37.9952) construction
  line L74 (70.2641, 37.9952) -> (70.2323, 37.9993) construction
  line L75 (70.2323, 37.9993) -> (70.2323, 34.8875) construction
  line L76 (70.2323, 34.8875) -> (68.2214, 38.8246) construction
  line L77 (68.2214, 38.8246) -> (68.1802, 38.9059) construction
  line L78 (68.1802, 38.9059) -> (67.9361, 39.6747) construction
  line L79 (67.9361, 39.6747) -> (67.9236, 39.7672) construction
  line L80 (67.9236, 39.7672) -> (68.0189, 39.6996) construction
  line L81 (68.0189, 39.6996) -> (68.3935, 39.6143) construction
  line L82 (68.3935, 39.6143) -> (68.9323, 39.7175) construction
  line L83 (68.9323, 39.7175) -> (69.5098, 40.0208) construction
  line L84 (69.5098, 40.0208) -> (70.0981, 40.4687) construction
  line L85 (70.0981, 40.4687) -> (70.6662, 41.0034) construction
  line L86 (70.6662, 41.0034) -> (71.1853, 41.5655) construction
  line L87 (71.1853, 41.5655) -> (71.6262, 42.1005) construction
  line L88 (71.6262, 42.1005) -> (71.88, 42.434) construction
  line L89 (71.88, 42.434) -> (71.9597, 42.5483) construction
  line L90 (71.9597, 42.5483) -> (72.5675, 43.4261) construction
  line L91 (72.5675, 43.4261) -> (74.1218, 46.2471) construction
  line L92 (74.1218, 46.2471) -> (75.642, 49.9608) construction
  line L93 (75.642, 49.9608) -> (76.5419, 53.4045) construction
  line L94 (76.5419, 53.4045) -> (76.8406, 55.5681) construction
  line L95 (76.8406, 55.5681) -> (76.8434, 56.2889) construction
  line L96 (76.8434, 56.2889) -> (76.8434, 56.435) construction
  line L97 (76.8434, 56.435) -> (76.8132, 57.8239) construction
  line L98 (76.8132, 57.8239) -> (76.8078, 57.9562) construction
  line L99 (76.8078, 57.9562) -> (76.7552, 57.2463) construction
  line L100 (76.7552, 57.2463) -> (76.3735, 55.134) construction
  line L101 (76.3735, 55.134) -> (75.4337, 51.9024) construction
  line L102 (75.4337, 51.9024) -> (73.9676, 48.4838) construction
  line L103 (73.9676, 48.4838) -> (72.519, 45.9039) construction
  line L104 (72.519, 45.9039) -> (71.9597, 45.0977) construction
  line L105 (71.9597, 45.0977) -> (71.8703, 44.971) construction
  line L106 (71.8703, 44.971) -> (71.5617, 44.6181) construction
  line L107 (71.5617, 44.6181) -> (71.0408, 44.1442) construction
  line L108 (71.0408, 44.1442) -> (70.4385, 43.7363) construction
  line L109 (70.4385, 43.7363) -> (69.7989, 43.4538) construction
  line L110 (69.7989, 43.4538) -> (69.1639, 43.3598) construction
  line L111 (69.1639, 43.3598) -> (68.5754, 43.5117) construction
  line L112 (68.5754, 43.5117) -> (68.0791, 43.9704) construction
  line L113 (68.0791, 43.9704) -> (67.7746, 44.5823) construction
  line L114 (67.7746, 44.5823) -> (67.7167, 44.7972) construction
  line L115 (67.7167, 44.7972) -> (66.74, 41.5577) construction
  line L116 (66.74, 41.5577) -> (66.657, 41.2323) construction
  line L117 (66.657, 41.2323) -> (66.2008, 39.7881) construction
  line L118 (66.2008, 39.7881) -> (65.6869, 38.578) construction
  line L119 (65.6869, 38.578) -> (65.5767, 38.3703) construction
  line L120 (65.5767, 38.3703) -> (63.7248, 41.0987) construction
  line L121 (59.1274, 36.9164) -> (59.2762, 36.7563) construction
  line L122 (60.1375, 41.0987) -> (59.1274, 36.9164) construction
  line L123 (59.1274, 36.9164) -> (60.1375, 41.0987) construction
  line L124 (60.1375, 41.0987) -> (58.1904, 38.2308) construction
  line L125 (61.0652, 35.7505) -> (61.9509, 40.717) construction
  line L126 (61.9509, 40.717) -> (62.9338, 35.8292) construction
  line L127 (62.9338, 35.8292) -> (61.9509, 40.717) construction
  line L128 (64.5625, 36.9024) -> (64.7002, 37.0611) construction
  line L129 (64.7002, 37.0611) -> (63.7248, 41.0987) construction
  line L130 (64.7002, 37.0611) -> (63.7248, 41.0987) construction
  line L131 (63.7248, 41.0987) -> (65.5767, 38.3703) construction
  line L132 (59.1274, 36.9164) -> (59.2018, 36.8363) construction
  line L133 (59.2018, 36.8363) -> (59.2762, 36.7563) construction
  line L134 (59.2762, 36.7563) -> (60.0646, 36.1516) construction
  line L135 (59.2762, 36.7563) -> (59.6704, 36.454) construction
  line L136 (60.0646, 36.1516) -> (60.894, 35.7889) construction
  line L137 (59.6704, 36.454) -> (60.0646, 36.1516) construction
  line L138 (60.0646, 36.1516) -> (60.4793, 35.9702) construction
  line L139 (60.894, 35.7889) -> (61.0652, 35.7505) construction
  line L140 (60.4793, 35.9702) -> (60.894, 35.7889) construction
  line L141 (60.894, 35.7889) -> (60.9796, 35.7697) construction
  line L142 (60.9796, 35.7697) -> (61.0652, 35.7505) construction
  spline S0 degree 4 poles (59.1274, 36.9164) (59.2018, 36.8363) (59.2762, 36.7563) (59.6704, 36.454) (60.0646, 36.1516) (60.4793, 35.9702) (60.894, 35.7889) (60.9796, 35.7697) (61.0652, 35.7505) knots 1 1 1 1 1 2 3 4 5 6 6 6 6 6
  line L143 (55.9732, 44.7972) -> (56.9488, 41.5577) construction
  line L144 (56.9488, 41.5577) -> (57.0357, 41.2143) construction
  line L145 (57.0357, 41.2143) -> (57.5221, 39.6984) construction
  line L146 (57.5221, 39.6984) -> (58.0718, 38.4447) construction
  line L147 (58.0718, 38.4447) -> (58.1904, 38.2308) construction
  line L148 (46.8754, 57.8239) -> (46.8823, 57.9562) projected
  line L149 (46.8823, 57.9562) -> (46.9331, 57.2478) projected
  line L150 (46.9331, 57.2478) -> (47.3149, 55.134) projected
  line L151 (47.3149, 55.134) -> (48.2547, 51.9024) projected
  line L152 (48.2547, 51.9024) -> (49.7197, 48.4838) projected
  line L153 (49.7197, 48.4838) -> (51.1693, 45.9052) projected
  line L154 (51.1693, 45.9052) -> (51.7301, 45.0977) projected
  line L155 (51.7301, 45.0977) -> (51.8185, 44.971) projected
  line L156 (51.8185, 44.971) -> (52.1272, 44.6181) projected
  line L157 (51.8185, 44.971) -> (51.1693, 45.9052)
  line L158 (52.1272, 44.6181) -> (52.6479, 44.1442) projected
  line L159 (52.6479, 44.1442) -> (53.2501, 43.7363) projected
  line L160 (53.2501, 43.7363) -> (53.8897, 43.4538) projected
  line L161 (53.8897, 43.4538) -> (54.5249, 43.3598) projected
  line L162 (54.5249, 43.3598) -> (55.1119, 43.5117) projected
  line L163 (55.1119, 43.5117) -> (55.6095, 43.9704) projected
  line L164 (55.6095, 43.9704) -> (55.9138, 44.5823) projected
  line L165 (55.9138, 44.5823) -> (55.9732, 44.7972) projected
  point P0 (0, 0)
  point P1 (56.461, 43.1775)
  point P2 (56.9923, 41.386)
  point P3 (57.2789, 40.4564)
  point P4 (57.7969, 39.0716)
  point P5 (58.1311, 38.3377)
  point P6 (46.9077, 57.602)
  point P7 (47.124, 56.1909)
  point P8 (47.7848, 53.5182)
  point P9 (48.9872, 50.1931)
  point P10 (50.4445, 47.1945)
  point P11 (51.9728, 44.7946)
  point P12 (51.4939, 45.4381)
  point P13 (52.3875, 44.3812)
  point P14 (52.949, 43.9402)
  point P15 (53.5699, 43.595)
  point P16 (54.2073, 43.4068)
  point P17 (54.8184, 43.4358)
  point P18 (55.3607, 43.7411)
  point P19 (55.7616, 44.2764)
  point P20 (55.9435, 44.6898)
  constraints: 24 coincident, 24 midpoint, 14 end point, 7 collinear, 3 other